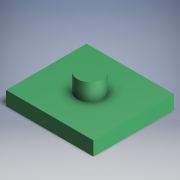
# Autodesk Inventor part: Camera
Saved by Autodesk Inventor 2018 (Build 220112000, 112)
## iProperties
Created: 2017-05-31
Part Number: Camera
Material: ABS Plastic
Document SubType Name: Modeling
Designer: Rishi
Density: 1.06 g/cm^3
Appearance: Smooth - White
Author: Rishi
Autodesk Inventor part; units mm, degrees
ref_plane "YZ Plane" through (0, 0, 0) normal (1, 0, 0) x (0, 1, 0)
ref_plane "XZ Plane" through (0, 0, 0) normal (0, 1, 0) x (-1, 0, 0)
ref_plane "XY Plane" through (0, 0, 0) normal (0, 0, 1) x (1, 0, 0)
sketch "Sketch1" plane through (0, 0, 0) normal (0, 1, 0) x (-1, 0, 0)
  line L0 (25, 23) -> (0, 23)
  line L1 (0, 23) -> (0, 0)
  line L2 (0, 0) -> (25, 0)
  line L3 (25, 0) -> (25, 23)
  dimension "d0" = 25
  dimension "d1" = 23
  constraints: 8 end point, 2 parallel, 1 horizontal, 1 perpendicular
  measures "d0" distance of L0.start L0.end
  measures "d1" distance of L2.end L0.start
extrude "Extrusion1" add sketch "Sketch1" along normal blind 4
sketch "Sketch2" plane through (0, 4, 0) normal (0, 1, 0) x (1, 0, 0)
  circle A0 centre (-12.5, -11.5) radius 3.615
  line L0 (-25, 0) -> (-25, -23) projected
  line L1 (-25, -23) -> (0, -23) projected
  point P0 (0, 0)
  dimension "d4" = 7.23
  dimension "d5" = 12.5
  dimension "d6" = 11.5
  constraints: 1 centre point
  measures "d4" diameter of A0
  measures "d5" distance from line of A0.centre L0
  measures "d6" distance from line of L1 A0.centre
extrude "Extrusion2" add sketch "Sketch2" along normal blind 5
body "Solid1"
